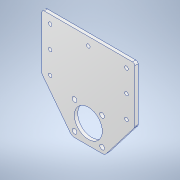
# Autodesk Inventor part: 関節4_側板
Saved by Autodesk Inventor 2021 (Build 250183000, 183)
## iProperties
Created: 2022-02-03
Part Number: 関節4_側板
Material: アルミニウム 6061
Document SubType Name: Modeling
Designer: hirohumi
Density: 2.7 g/cm^3
Appearance: アルミニウム - フラット
Author: hirohumi
Autodesk Inventor part; units mm, degrees
ref_plane "YZ Plane" through (0, 0, 0) normal (1, 0, 0) x (0, 1, 0)
ref_plane "XZ Plane" through (0, 0, 0) normal (0, 1, 0) x (-1, 0, 0)
ref_plane "XY Plane" through (0, 0, 0) normal (0, 0, 1) x (1, 0, 0)
sketch "スケッチ1" plane through (0, 0, 0) normal (0, 0, 1) x (1, 0, 0)
  circle A0 centre (-34.3, -20) radius 1.6
  circle A1 centre (-34.3, 0) radius 1.6
  circle A2 centre (-34.3, -40) radius 1.6
  circle A3 centre (34.3, -20) radius 1.6
  circle A4 centre (34.3, 0) radius 1.6
  circle A5 centre (34.3, -40) radius 1.6
  circle A6 centre (0, 0) radius 1.6
  circle A7 centre (0, 0) radius 50 construction
  circle A8 centre (0, -60.2) radius 10 construction
  circle A9 centre (0, -60.2) radius 12.55
  circle A10 centre (-12.3744, -47.8256) radius 2.15
  circle A11 centre (-12.3744, -72.5744) radius 2.15
  circle A12 centre (12.3744, -72.5744) radius 2.15
  circle A13 centre (12.3744, -47.8256) radius 2.15
  line L0 (12.3744, -47.8256) -> (-12.3744, -47.8256) construction
  line L1 (-12.3744, -47.8256) -> (-12.3744, -72.5744) construction
  line L2 (-12.3744, -72.5744) -> (12.3744, -72.5744) construction
  line L3 (12.3744, -72.5744) -> (12.3744, -47.8256) construction
  line L4 (12.3744, -47.8256) -> (-12.3744, -72.5744) construction
  line L5 (-12.3744, -47.8256) -> (12.3744, -72.5744) construction
  line L6 (-41.8, 7.5) -> (41.8, 7.5)
  line L7 (41.8, 7.5) -> (41.8, -42.5528)
  line L8 (41.8, -42.5528) -> (16.3361, -75.6247)
  line L9 (-41.8, 7.5) -> (-41.8, -42.5528)
  line L10 (-41.8, -42.5528) -> (-16.3361, -75.6247)
  arc A14 (-16.3361, -75.6247) -> (-12.3744, -77.5744) centre (-12.3744, -72.5744) ccw
  arc A15 (12.3744, -77.5744) -> (16.3361, -75.6247) centre (12.3744, -72.5744) ccw
  line L11 (-12.3744, -77.5744) -> (12.3744, -77.5744)
  dimension "d0" = 3.2
  dimension "d1" = 3.2
  dimension "d2" = 3.2
  dimension "d3" = 20
  dimension "d4" = 20
  dimension "d5" = 3.2
  dimension "d6" = 3.2
  dimension "d7" = 3.2
  dimension "d8" = 20
  dimension "d9" = 20
  dimension "d10" = 68.6
  dimension "d11" = 34.3
  dimension "d12" = 3.2
  dimension "d13" = 100
  dimension "d14" = 20
  dimension "d15" = 60.2
  dimension "d16" = 25.1
  dimension "d17" = 4.3
  dimension "d18" = 4.3
  dimension "d19" = 4.3
  dimension "d20" = 4.3
  dimension "d21" = 35
  dimension "d22" = 5
  dimension "d23" = 7.5
  dimension "d24" = 7.5
  dimension "d25" = 7.5
  dimension "d26" = 7.5
  dimension "d27" = 7.5
  constraints: 24 end point, 16 centre point, 8 coincident, 5 vertical alignment, 4 point on circle, 4 tangent, 3 horizontal, 3 perpendicular, 2 horizontal alignment, 2 midpoint, 2 parallel, 1 vertical
  measures "d0" diameter of A0
  measures "d1" diameter of A1
  measures "d2" diameter of A2
  measures "d3" distance of A0.centre A1.centre
  measures "d4" distance of A2.centre A0.centre
  measures "d5" diameter of A3
  measures "d6" diameter of A4
  measures "d7" diameter of A5
  measures "d8" distance of A3.centre A4.centre
  measures "d9" distance of A5.centre A3.centre
  measures "d10" distance of A3.centre A0.centre
  measures "d11" horizontal distance of point (0, 0) A0.centre
  measures "d12" diameter of A6
  measures "d13" diameter of A7
  measures "d14" diameter of A8
  measures "d15" distance of A8.centre point (0, 0)
  measures "d16" diameter of A9
  measures "d17" diameter of A10
  measures "d18" diameter of A11
  measures "d19" diameter of A12
  measures "d20" diameter of A13
  measures "d21" distance of L0.end L2.end
  measures "d22" radius of A14
  measures "d23" distance from line of A1.centre L9
  measures "d24" distance from line of A1.centre L6
  measures "d25" distance from line of A4.centre L7
  measures "d26" distance from line of A2.centre L10
  measures "d27" distance from line of L8 A5.centre
extrude "押し出し1" add sketch "スケッチ1" along normal blind 3
fillet "フィレット1" radius 2 4 edges at (-41.8, 7.5, 1.5) (41.8, 7.5, 1.5) (41.8, -42.5528, 1.5) (-41.8, -42.5528, 1.5)
equation "\"d11\" = 0.5 * d10"
